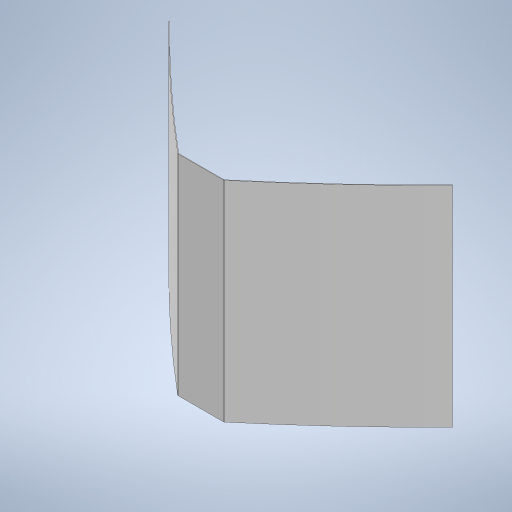
# Autodesk Inventor part: МОО 030 лист брюхо 1
Saved by Autodesk Inventor 2024.2 (Build 282272000, 272)
## iProperties
Created: 2024-04-28
Part Number: МОО 030 лист брюхо 1
Material: Stainless Steel
Document SubType Name: Sheet Metal
Designer: admin
Density: 8 g/cm^3
Flat Pattern Width: 100 cm
Flat Pattern Length: 176.414 cm
Flat Pattern Area: 17641.4 cm^2
Sheet Metal Rule: Default_mm
Sheet Metal Width: 1000,000 mm
Sheet Metal Length: 1764,143 mm
Sheet Metal Area: 1764143,085 mm^2
Appearance: Default
Mass: 43869.2 g
Surface Area: 36727.4 cm^2
Volume: 5483.66 cm^3
Author: admin
Autodesk Inventor part; units mm, degrees
note: some values were not read from the file. Chosen so that the rebuilt part matches the saved one: flange form of "Plate1".
ref_plane "YZ Plane" through (0, 0, 0) normal (1, 0, 0) x (0, 1, 0)
ref_plane "XZ Plane" through (0, 0, 0) normal (0, 1, 0) x (-1, 0, 0)
ref_plane "XY Plane" through (0, 0, 0) normal (0, 0, 1) x (1, 0, 0)
sketch "Sketch1" plane through (0, 0, 0) normal (0, 0, 1) x (1, 0, 0)
  line L0 (-750, 0) -> (750, 0) construction
  line L1 (750, 0) -> (750, -2100) construction
  line L2 (750, -2100) -> (110, -2700) construction
  line L3 (107.8152, -2700) -> (-107.8152, -2700)
  line L4 (-110, -2700) -> (-750, -2100) construction
  line L5 (-750, -2100) -> (-750, 0) construction
  arc A0 (745.2369, 0.4471) -> (-745.2369, 0.4471) centre (0, -7964.7662) ccw construction
  arc A1 (-750.6265, -4.7429) -> (-777.5832, -235) centre (7180.7944, -1050) ccw construction
  arc A2 (-777.5832, -235) -> (-750.1285, -2099.0286) centre (7180.7944, -1050) ccw construction
  arc A3 (750.1285, -2099.0286) -> (777.5832, -235) centre (-7180.7944, -1050) ccw construction
  arc A4 (777.5832, -235) -> (750.6265, -4.7429) centre (-7180.7944, -1050) ccw construction
  line L6 (-777.5832, -235) -> (777.5832, -235) construction
  arc A5 (-749.3229, -2100.7083) -> (-677.5699, -2174.8011) centre (5033.2984, 3427.5183) ccw construction
  line L7 (-750, -2100) -> (750, -2100) construction
  line L8 (-547.1729, -2035.7109) -> (-801.0834, -2306.5488) construction
  arc A6 (-677.5699, -2174.8011) -> (-111.6739, -2698.5946) centre (5033.2984, 3427.5183) ccw
  arc A7 (-745.2369, 0.4471) -> (-750.6265, -4.7429) centre (-744.6779, -5.5268) ccw construction
  arc A8 (750.6265, -4.7429) -> (745.2369, 0.4471) centre (744.6779, -5.5268) ccw construction
  arc A9 (-750.1285, -2099.0286) -> (-749.3229, -2100.7083) centre (-747.1545, -2098.6352) ccw construction
  arc A10 (111.6739, -2698.5946) -> (677.5699, -2174.8011) centre (-5033.2984, 3427.5183) ccw
  line L9 (553.8195, -2042.8006) -> (794.4368, -2299.4591) construction
  arc A11 (677.5699, -2174.8011) -> (749.3229, -2100.7083) centre (-5033.2984, 3427.5183) ccw construction
  arc A12 (749.3229, -2100.7083) -> (750.1285, -2099.0286) centre (747.1545, -2098.6352) ccw construction
  arc A13 (-111.6739, -2698.5946) -> (-107.8152, -2700) centre (-107.8152, -2694) ccw
  arc A14 (107.8152, -2700) -> (111.6739, -2698.5946) centre (107.8152, -2694) ccw
  point P0 (0, 0)
  point P1 (0, 0)
  point P2 (0, 0)
  point P3 (0, -2700)
  point P4 (-674.1281, -2171.1299)
  point P5 (674.1281, -2171.1299)
  dimension "d19" = 1500
  dimension "d20" = 2100
  dimension "d21" = 220
  dimension "d22" = 2700
  dimension "d23" = 8000
  dimension "d24" = 8000
  dimension "d25" = 8000
  dimension "d26" = 235
  dimension "d27" = 8000
  dimension "d28" = 104
  dimension "d29" = 6
  dimension "d30" = 3
  dimension "d31" = 8000
  dimension "d32" = 104
  dimension "d33" = 6
  measures "d19" distance of L0.end L0.start
  measures "d20" distance of L2.start L0.end
  measures "d21" distance of L2.end L4.start
  measures "d22" vertical distance of point (0, -2700) L0.start
  measures "d23" radius of A0
  measures "d24" radius of A1
  measures "d25" radius of A3
  measures "d26" distance between parallel lines of L0 L6
  measures "d27" radius of A5
  measures "d28" distance of L4.end point (-674.128, -2171.13)
  measures "d29" radius of A7
  measures "d30" radius of A9
  measures "d31" radius of A10
  measures "d32" distance of L2.start point (674.128, -2171.13)
  measures "d33" radius of A13
contour flange "Contour Flange1" sketch "Sketch1" thickness 3 bend radius 3 width 1000 along (0, 0, 1) mid plane no both sides no wall seen from (-400.9365, -2443.52, 0) lies toward (0.6792794, 0.7338798, 0) curves A6 A13 L3 A14 A10
bend "Bend1"
corner "Corner1"
equation "\"d19\" = Бак_ширина_общая"
equation "\"d20\" = Бак_высота_до_конуса"
equation "\"d21\" = Бак_брюхо_ширина_полки"
equation "\"d22\" = Бак_высота_общая"
equation "\"d23\" = Бак_радиус_стенок_общий"
equation "\"d24\" = Бак_радиус_стенок_общий"
equation "\"d25\" = Бак_радиус_стенок_общий"
equation "\"d26\" = Бак_спина_длина_фланцев"
equation "\"d27\" = Бак_радиус_стенок_общий"
equation "\"d28\" = Бак_борт_длина_фланца"
equation "\"d29\" = d41 + d42"
equation "\"d30\" = d41"
equation "\"d31\" = Бак_радиус_стенок_общий"
equation "\"d32\" = Бак_борт_длина_фланца"
equation "\"d33\" = Thickness + BendRadius"
equation "\"d7\" = Thickness"
equation "\"d8\" = BendReliefWidth"
equation "\"d9\" = BendReliefDepth"
equation "\"d10\" = MinimumRemnant"
equation "\"d11\" = TransitionRadius"
equation "\"d13\" = BendRadius"
equation "\"d15\" = CornerReliefSize"
equation "\"d16\" = GapSize"
equation "\"d17\" = JacobiRadiusSize"
equation "\"BendRadius\" = Thickness"
equation "\"BendReliefWidth\" = Thickness"
equation "\"BendReliefDepth\" = 0.5 * Thickness"
equation "\"CornerReliefSize\" = 4 * Thickness"
equation "\"MinimumRemnant\" = 2 * Thickness"
equation "\"TransitionRadius\" = BendRadius"
equation "\"JacobiRadiusSize\" = BendRadius"
equation "\"GapSize\" = Thickness"
equation "\"d42\" = d41"
equation "\"Бак_ширина_общая\" = 1500"
equation "\"Бак_высота_до_конуса\" = 2100"
equation "\"Бак_брюхо_ширина_полки\" = 220"
equation "\"Бак_радиус_стенок_общий\" = 8000"
equation "\"Бак_спина_длина_фланцев\" = 235"
equation "\"d41\" = 3"
equation "\"Thickness\" = 3"
equation "\"Бак_высота_общая\" = 2700"
equation "\"Бак_борт_длина_фланца\" = 104"
body "Solid1"
